Bearing (Autodesk Fusion 360 design; units mm, degrees)
part number: 2026-09-27-15-55-38-168
part number: 2026-09-27-16-09-37-496
part number: 2026-09-27-16-09-37-513
part number: 2026-09-27-16-09-37-520
part number: 2026-09-27-16-09-37-525
part number: 2026-09-27-16-09-37-532
part number: 2026-09-27-16-09-37-536
part number: 2026-09-27-16-09-37-543
part number: 2026-09-27-16-09-37-548
part number: 2026-09-27-16-09-37-554
part number: 2026-09-27-16-09-37-559
part number: 2026-09-27-16-09-37-564
Autodesk Fusion 360 part; units mm, degrees
note: some values were not read from the file. Set by a fixed rule: which sketch regions a step uses.
sketch "Sketch1" plane through (0, 0, 0) normal (0, 1, 0) x (1, 0, 0)
  circle A0 centre (-125, -75) radius 20
  line L0 (-100, -85) -> (-150, -85)
  line L1 (-150, -85) -> (-150, -105)
  line L2 (-150, -105) -> (-100, -105)
  line L3 (-100, -105) -> (-100, -85)
  line L4 (-100, -85) -> (-150, -105) construction
  line L5 (-150, -85) -> (-100, -105) construction
  line L6 (-100, -45) -> (-150, -45)
  line L7 (-150, -45) -> (-150, -65)
  line L8 (-150, -65) -> (-100, -65)
  line L9 (-100, -65) -> (-100, -45)
  line L10 (-100, -45) -> (-150, -65) construction
  line L11 (-150, -45) -> (-100, -65) construction
  line L12 (-125, -105) -> (-125, -5)
  line L13 (-125, -5) -> (-80, -5)
  point P0 (-125, -95)
  point P1 (-125, -55)
  dimension "d1" = 50
  dimension "d2" = 20
  dimension "d3" = 100
  constraint horizontal L0
  constraint perpendicular L0 L1
  constraint parallel L0 L2
  constraint parallel L1 L3
  constraint coincident L4 P0
  constraint coincident L5 P0
  constraint coincident A0 P0
  constraint horizontal L6
  constraint perpendicular L6 L7
  constraint parallel L6 L8
  constraint parallel L7 L9
  constraint coincident L10 P1
  constraint coincident L11 P1
  constraint coincident A0 P1
  constraint midpoint L2 L12.start
  constraint perpendicular L2 L12
  constraint perpendicular L12 L13
  measures "d1" distance of L1.end L2.end
  measures "d2" distance of L0.end L1.end
  measures "d3" distance of L12.start L12.end
revolve "Revolve1" add sketch "Sketch1" angle 360 about axis through (-125, 0, 5) along (1, 0, 0) contours A0 L6 L8 L9 L12 | A0 L0 L2 L3 L12 | A0 L6 L7 L8 L12 | A0 L0 L1 L2 L12 makes body 1 at (-133.3333, 4.9846, 104.8757) makes body 2 at (-108.1995, 5.8893, 63.8551)
revolve "Revolve2" add sketch "Sketch1" angle 360 about axis through (-125, 0, 105) along (0, 0, -1) separate body contours A0 L0 L8 L12 | A0 L8 L12 | A0 L0 L12 picked at (-118.3333, -75) picked at (-124.0064, -58.4078) picked at (-124.0064, -91.5922) makes body 3
pattern_circular "C-Pattern1" count 8 over 360 about axis through (-125, 0, 5) along (1, 0, 0) of bodies 3 makes body 4 at (-109.3306, -43.3121, 43.7173) makes body 5 at (-109.3306, -58.0036, 1.751) makes body 6 at (-109.3306, -38.7173, -38.3121) makes body 7 at (-109.3306, 3.249, -53.0036) makes body 8 at (-109.3306, 43.3121, -33.7173) makes body 9 at (-109.3306, 58.0036, 8.249) makes body 10 at (-109.3306, 38.7173, 48.3121)
sketch "Sketch2" plane through (0, 0, 0) normal (1, 0, 0) x (0, 1, 0)
  circle A0 through (72.5, 5, -120) (-36.25, 67.7868, -120) (-36.25, -57.7868, -120)
  circle A1 through (67.5, 5, -120) (-33.75, 63.4567, -120) (-33.75, -53.4567, -120)
  dimension "d8" = 145
  dimension "d9" = 135
sketch "Sketch2 (curves -120 mm off its plane)" plane through (-120, 0, 0) normal (1, 0, 0) x (0, 1, 0)
  circle A0 centre (0, 5) radius 72.5
  circle A1 centre (0, 5) radius 67.5
extrude "Extrude1" add sketch "Sketch2 (curves -120 mm off its plane)" against normal blind 25 separate body makes body 11
combine "Combine1" operation cut target body 10 tool bodies 3 4 5 6 7 8 9 keep tools
combine "Combine2" operation cut target body 11 tool bodies 6 4 7 5 10 9 8 3 keep tools
shell "Shell1" thickness 2 removed faces 3 at (-145, 70.3121, -1.9553) at (-135.1172, 27.3451, 72.1453) at (-135.8924, 25.4618, 67.5136) on bodies 11
mirror "Mirror1" about plane through (-120, 0, 0) normal (1, 0, 0) of bodies 11 merged
copy_body "Body->Comp1" bodies 1 removing the originals makes body 12 in component "Component"
copy_body "Body->Comp2" bodies 2 removing the originals makes body 13 in component "Component'"
copy_body "Body->Comp3" bodies 3 removing the originals makes body 14 in component "Component''"
copy_body "Body->Comp4" bodies 4 removing the originals makes body 15 in component "Component'''"
copy_body "Body->Comp5" bodies 5 removing the originals makes body 16 in component "Component''''"
copy_body "Body->Comp6" bodies 6 removing the originals makes body 17 in component "Component'''''"
copy_body "Body->Comp7" bodies 7 removing the originals makes body 18 in component "Component''''''"
copy_body "Body->Comp8" bodies 8 removing the originals makes body 19 in component "Component'''''''"
copy_body "Body->Comp9" bodies 9 removing the originals makes body 20 in component "Component''''''''"
copy_body "Body->Comp10" bodies 10 removing the originals makes body 21 in component "Component'''''''''"
copy_body "Body->Comp11" bodies 11 removing the originals makes body 22 in component "Component''''''''''"
component "Component" placed x (1, 0, 0) y (0, 1, 0) z (0, 0, 1) at (0, 0, 0)
component "Component'" placed x (1, 0, 0) y (0, 1, 0) z (0, 0, 1) at (0, 0, 0)
component "Component''" placed x (1, 0, 0) y (0, 1, 0) z (0, 0, 1) at (0, 0, 0)
component "Component'''" placed x (1, 0, 0) y (0, 1, 0) z (0, 0, 1) at (0, 0, 0)
component "Component''''" placed x (1, 0, 0) y (0, 1, 0) z (0, 0, 1) at (0, 0, 0)
component "Component'''''" placed x (1, 0, 0) y (0, 1, 0) z (0, 0, 1) at (0, 0, 0)
component "Component''''''" placed x (1, 0, 0) y (0, 1, 0) z (0, 0, 1) at (0, 0, 0)
component "Component'''''''" placed x (1, 0, 0) y (0, 1, 0) z (0, 0, 1) at (0, 0, 0)
component "Component''''''''" placed x (1, 0, 0) y (0, 1, 0) z (0, 0, 1) at (0, 0, 0)
component "Component'''''''''" placed x (1, 0, 0) y (0, 1, 0) z (0, 0, 1) at (0, 0, 0)
component "Component''''''''''" placed x (1, 0, 0) y (0, 1, 0) z (0, 0, 1) at (0, 0, 0)
